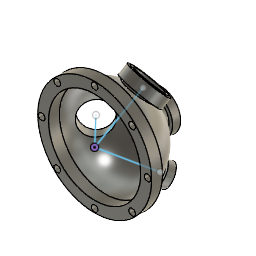
H1 (Autodesk Fusion 360 design; units mm, degrees)
part number: 2026-06-30-06-54-06-538
Autodesk Fusion 360 part; units mm, degrees
note: some values were not read from the file. Set by a fixed rule: which sketch regions a step uses.
sketch "Sketch8" plane through (0, 0, 0) normal (0, 0, 1) x (1, 0, 0)
  line L0 (-63.5, 0.0319) -> (-78.5, 0.0396)
  line L1 (-63.5, 0.0319) -> (-63.4923, 15.0319)
  line L2 (-63.4923, 15.0319) -> (-78.4923, 15.0396)
  line L3 (-78.5, 0.0396) -> (-78.4923, 15.0396)
  line L4 (0, 0) -> (0, 73.5) construction
  arc A0 (0, 73.5) -> (-63.4923, 15.0319) centre (-1.1724, 11.065) ccw
  arc A1 (0, 76.5005) -> (-66.5, 15) centre (-1.1724, 11.065) ccw
  line L5 (0, 73.5) -> (0, 76.5005)
  dimension "d33" = 63.5
  dimension "d34" = 15
  dimension "d35" = 15
  dimension "d36" = 15
  dimension "d37" = 73.5
  dimension "d39" = 3
  constraint perpendicular L0 L1
  constraint perpendicular L1 L2
  constraint coincident L4.start origin
  constraint vertical L4
  measures "d33" distance of L4.start L0.start
  measures "d34" distance of L0.start L0.end
  measures "d35" distance of L0.start L1.end
  measures "d36" distance of L1.end L2.end
  measures "d37" distance of L4.start L4.end
revolve "Revolve3" add sketch "Sketch8" angle 360 about axis through (0, 0, 0) along (0, 1, 0) makes body 1
sketch "Sketch11" plane through (0, 0, 0) normal (0, 1, 0) x (1, 0, 0)
  circle A0 centre (-73, 0) radius 4.5
  dimension "d41" = 9
  measures "d41" diameter of A0
extrude "Extrude5" cut sketch "Sketch11" along normal blind 27 bodies 1
pattern_circular "C-Pattern1" count 8 over 360 about axis through (0, 11.065, 0) along (0, 1, 0) of "Extrude5"
ref_plane "WorkPlane1" through (0, 80, 0) normal (0, 1, 0) x (0, 0, 1)
sketch "Sketch12" plane through (0, 80, 0) normal (0, 1, 0) x (1, 0, 0)
  circle A0 centre (0, 0) radius 27.5
  dimension "d47" = 55
  constraint coincident A0.centre origin
  measures "d47" diameter of A0
extrude "Extrude6" add sketch "Sketch12" along normal blind 12 separate body makes body 2
sketch "Sketch13" plane through (0, 80, 0) normal (0, -1, 0) x (1, 0, 0)
  circle A0 centre (0, 0) radius 27.5
  circle A1 centre (0, 0) radius 22.5
  dimension "d51" = 45
  measures "d51" diameter of A1
extrude "Extrude7" add sketch "Sketch13" along normal blind 9 contours A1 bodies 1 2
sketch "Sketch14" plane through (0, 71, 0) normal (0, -1, 0) x (1, 0, 0)
  circle A0 centre (0, 0) radius 18.7024
  circle A1 centre (0, 0) radius 20
  dimension "d54" = 40
  constraint concentric A0 A1
  measures "d54" diameter of A1
extrude "Extrude8" cut sketch "Sketch14" against normal blind 30 contours A0 bodies 1
chamfer "Chamfer1" distance 3 angle 15 1 edges at (-25.639, 92, 9.9444) measured on face at (24.3954, 92, 2.2954) on bodies 1
sketch "Sketch15" plane through (0, 0, 0) normal (0, 1, 0) x (1, 0, 0)
ref_plane "WorkPlane2" through (9.0587, 0, 33.8074) normal (-0.965926, 0, 0.258819) x (0.258819, 0, 0.965926)
sketch "Sketch16" plane through (0, 0, 0) normal (-0.965926, 0, 0.258819) x (0.258819, 0, 0.965926)
  line L0 (0, 0) -> (53.033, 53.033)
  dimension "d64" = 75
  constraint coincident L0.start origin
  measures "d64" distance of L0.start L0.end
ref_plane "WorkPlane3" through (24.7487, 0, -24.7487) normal (0.707107, 0, 0.707107) x (0.707107, 0, -0.707107)
sketch "Sketch17" plane through (0, 0, 0) normal (0.707107, 0, 0.707107) x (0.707107, 0, -0.707107)
  line L0 (0, 0) -> (53.033, 53.033)
  dimension "d67" = 75
  constraint coincident L0.start origin
  measures "d67" distance of L0.start L0.end
ref_plane "WorkPlane4" through (-33.8074, 0, -9.0587) normal (0.258819, 0, -0.965926) x (-0.965926, 0, -0.258819)
sketch "Sketch18" plane through (0, 0, 0) normal (0.258819, 0, -0.965926) x (-0.965926, 0, -0.258819)
  line L0 (0, 0) -> (53.033, 53.033)
  dimension "d70" = 75
  constraint coincident L0.start origin
  measures "d70" distance of L0.start L0.end
ref_plane "WorkPlane5" through (-51.226, 53.033, -13.726) normal (-0.683013, 0.707107, -0.183013) x (-0.719255, -0.694747, 0)
sketch "Sketch19" plane through (-51.226, 53.033, -13.726) normal (-0.683013, 0.707107, -0.183013) x (-0.719255, -0.694747, 0)
  circle A0 centre (0, 0) radius 27.5
  dimension "d73" = 55
  constraint coincident A0.centre origin
  measures "d73" diameter of A0
extrude "Extrude9" add sketch "Sketch19" along normal blind 10 separate body makes body 3
sketch "Sketch20" plane through (-58.0561, 60.1041, -15.5561) normal (-0.683013, 0.707107, -0.183013) x (-0.719255, -0.694747, 0)
  circle A0 centre (0, 0) radius 27.5
  circle A1 centre (0, 0) radius 20
  dimension "d76" = 40
  constraint concentric A0 A1
  measures "d76" diameter of A1
extrude "Extrude10" cut sketch "Sketch20" against normal blind 65 contours A1 bodies 1 3
sketch "Sketch21" plane through (-51.226, 53.033, -13.726) normal (0.683013, -0.707107, 0.183013) x (0.719255, 0.694747, 0)
  circle A0 centre (0, 0) radius 20
  circle A1 centre (0, 0) radius 27.5
  circle A2 centre (0, 0) radius 22.5
  dimension "d79" = 45
  constraint coincident A0.centre A1.centre
  measures "d79" diameter of A2
extrude "Extrude11" add sketch "Sketch21" along normal blind 5 contours A2 bodies 1 3
extrude "Extrude12" add 1 faces at (-46.739, 45.0621, -33.9482) along direction (0.683013, -0.707107, 0.183013) blind 3 on bodies 1 bodies 1
chamfer "Chamfer2" distance 3 angle 15 1 edges at (-38.3507, 76.6077, -25.3325) measured on face at (-75.6102, 42.5476, -17.8761) on bodies 1
ref_plane "WorkPlane6" through (13.726, 53.033, 51.226) normal (0.183013, 0.707107, 0.683013) x (-0.9681, 0.250563, 0)
sketch "Sketch22" plane through (13.726, 53.033, 51.226) normal (0.183013, 0.707107, 0.683013) x (-0.9681, 0.250563, 0)
  circle A0 centre (0, 0) radius 27.5
  dimension "d87" = 55
  constraint coincident A0.centre origin
  measures "d87" diameter of A0
extrude "Extrude13" add sketch "Sketch22" along normal blind 10 separate body makes body 4
sketch "Sketch23" plane through (13.726, 53.033, 51.226) normal (-0.183013, -0.707107, -0.683013) x (0.9681, -0.250563, 0)
  circle A0 centre (0, 0) radius 27.5
  circle A1 centre (0, 0) radius 22.5
  circle A2 centre (0, 0) radius 20 construction
  dimension "d90" = 45
  dimension "d91" = 40
  constraint coincident A0.centre A1.centre
  measures "d90" diameter of A1
  measures "d91" diameter of A2
extrude "Extrude14" add sketch "Sketch23" along normal blind 5 bodies 1 4
sketch "Sketch25" plane through (15.5561, 60.1041, 58.0561) normal (0.183013, 0.707107, 0.683013) x (-0.9681, 0.250563, 0)
  circle A0 centre (0, 0) radius 27.5
  circle A1 centre (0, 0) radius 20
  dimension "d98" = 40
  constraint coincident A0.centre A1.centre
  measures "d98" diameter of A1
extrude "Extrude17" cut sketch "Sketch25" against normal blind 55 contours A1 bodies 1
sketch "Sketch26" plane through (15.5561, 60.1041, 58.0561) normal (0.183013, 0.707107, 0.683013) x (-0.9681, 0.250563, 0)
  circle A0 centre (0, 0) radius 20
  circle A1 centre (0, 0) radius 27.5
  circle A2 centre (0, 0) radius 22.5
  dimension "d101" = 45
  constraint concentric A0 A2
  measures "d101" diameter of A2
extrude "Extrude18" add sketch "Sketch26" against normal blind 15 contours A2 bodies 1
sketch "Sketch27" plane through (12.8109, 49.4975, 47.8109) normal (-0.183013, -0.707107, -0.683013) x (0.9681, -0.250563, 0)
  spline S0 degree 3 poles (11.1154, -25.1535) (12.0084, -24.5146) (12.8756, -23.7937) (15.124, -21.6156) (16.368, -20.0161) (17.8114, -17.6117) (18.2935, -16.6837) (19.1172, -14.7675) (19.4589, -13.7793) (19.9981, -11.8432) (20.2329, -10.7056) (20.3754, -9.5517) (20.376, -9.5467) (20.3766, -9.5418) knots -4.64367 -4.64367 -4.64367 -4.64367 -4.332361 -4.332361 -3.77663 -3.77663 -3.491037 -3.491037 -3.205444 -3.205444 -2.888104 -2.888104 -2.886739 -2.886739 -2.886739 -2.886739
  arc A0 (11.1154, -25.1535) -> (-24.9936, -11.4704) centre (0, 0) ccw
  spline S1 degree 3 poles (-21.5829, 6.3583) (-21.5857, 6.3541) (-21.5886, 6.35) (-22.2466, 5.3914) (-22.8247, 4.384) (-23.7039, 2.5767) (-24.103, 1.6102) (-24.756, -0.3707) (-25.01, -1.385) (-25.5225, -4.1422) (-25.6509, -6.1645) (-25.4106, -9.2856) (-25.2389, -10.4002) (-24.9936, -11.4704) knots 2.886739 2.886739 2.886739 2.886739 2.888104 2.888104 3.205444 3.205444 3.491037 3.491037 3.77663 3.77663 4.332361 4.332361 4.64367 4.64367 4.64367 4.64367
  spline S2 degree 3 poles (-15.9564, 12.058) (-16.1019, 11.955) (-16.2463, 11.8503) (-17.5334, 10.894) (-18.5933, 9.9312) (-20.2007, 8.2053) (-20.9299, 7.3082) (-21.5829, 6.3583) knots 2.13017 2.13017 2.13017 2.13017 2.179197 2.179197 2.570764 2.570764 2.886739 2.886739 2.886739 2.886739
  arc A1 (19.9403, -1.5446) -> (-15.9564, 12.058) centre (0, 0) ccw
  spline S3 degree 3 poles (20.3766, -9.5418) (20.5171, -8.3976) (20.5655, -7.2425) (20.5056, -4.8848) (20.3498, -3.4614) (20.0198, -1.8923) (19.981, -1.7181) (19.9403, -1.5446) knots -2.886739 -2.886739 -2.886739 -2.886739 -2.570764 -2.570764 -2.179197 -2.179197 -2.13017 -2.13017 -2.13017 -2.13017
  circle A2 centre (0, 0) radius 22.5
  dimension "d104" = 45
  constraint concentric A0 A2
  measures "d104" diameter of A2
extrude "Extrude19" add sketch "Sketch27" along normal blind 3 contours S2 A1 S3 A2 picked at (21.567, -1.6058) bodies 1
chamfer "Chamfer3" distance 3 angle 15 1 edges at (42.0791, 60.2554, 50.7926) measured on face at (-8.0714, 67.8842, 56.3324) on bodies 1
ref_plane "WorkPlane7" through (37.5, 53.033, -37.5) normal (0.5, 0.707107, -0.5) x (-0.816497, 0.57735, 0)
sketch "Sketch28" plane through (37.5, 53.033, -37.5) normal (0.5, 0.707107, -0.5) x (-0.816497, 0.57735, 0)
  circle A0 centre (0, 0) radius 15
  dimension "d110" = 30
  constraint coincident A0.centre origin
  measures "d110" diameter of A0
extrude "Extrude20" add sketch "Sketch28" along normal blind 10 separate body makes body 5
sketch "Sketch29" plane through (42.5, 60.1041, -42.5) normal (0.5, 0.707107, -0.5) x (-0.816497, 0.57735, 0)
  circle A0 centre (0, 0) radius 15
  circle A1 centre (0, 0) radius 8
  dimension "d113" = 16
  constraint concentric A0 A1
  measures "d113" diameter of A1
extrude "Extrude21" cut sketch "Sketch29" against normal blind 70 contours A1 bodies 1 5
sketch "Sketch30" plane through (42.5, 60.1041, -42.5) normal (0.5, 0.707107, -0.5) x (-0.816497, 0.57735, 0)
  circle A0 centre (0, 0) radius 8
  circle A1 centre (0, 0) radius 15
  circle A2 centre (0, 0) radius 9.5
  dimension "d116" = 19
  constraint concentric A0 A2
  measures "d116" diameter of A2
extrude "Extrude22" add sketch "Sketch30" against normal blind 13 contours A2 bodies 1 5
chamfer "Chamfer4" distance 3 angle 15 1 edges at (52.3528, 49.8155, -47.1975) measured on face at (31.9882, 67.0807, -43.1454) on bodies 1
equation "chamber_ID = 100 mm" comment "Spherical chamber inner diameter"
equation "wall_thk = 3 mm" comment "Shell wall thickness"
equation "chamber_OD = chamber_ID + 2 * wall_thk" comment "Driven outer diameter"
equation "mouth_dia = 127 mm" comment "Hemisphere mouth opening (5 in)"
equation "flange_face_thk = 8 mm" comment "ISO-F flange ring thickness"
equation "flange_OD = 160 mm" comment "ISO-F flange outer diameter"
equation "bolt_circle_dia = 145 mm" comment "8-bolt pattern circle diameter"
equation "bolt_hole_dia = 8.4 mm" comment "M8 clearance hole"
equation "hv_boss_dia = 40 mm" comment "HV feedthrough housing OD (top pole)"
equation "kf40_boss_dia = 50.5 mm" comment "KF-40 small-end clamp diameter"
equation "kf25_boss_dia = 33.5 mm" comment "KF-25 small-end clamp diameter"
equation "kf16_boss_dia = 20.5 mm" comment "KF-16 small-end clamp diameter"
equation "port_stub_len = 25 mm" comment "Weld-neck stub length for all ports"
equation "atmo_lat = 55 deg" comment "Atmo/vent port latitude from north pole"
equation "atmo_az = 0 deg" comment "Atmo/vent port azimuth"
equation "maint_lat = 55 deg" comment "Maintenance port latitude from north pole"
equation "maint_az = 180 deg" comment "Maintenance port azimuth"
